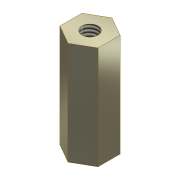
# Autodesk Inventor part: 黄銅スペーサー（六角）_ASB-2613.5E
Saved by Autodesk Inventor 2016 (Build 200138000, 138)
## iProperties
Created: 2016-08-20
Part Number: 黄銅スペーサー（六角）_ASB-2613.5E
Material: 真鍮、ソフト イエロー
Document SubType Name: Modeling
Designer: NN
Mass: 2.07468 g
Surface Area: 3.5973 cm^2
Volume: 0.244944 cm^3
Density: 8.47 g/cm^3
Appearance: ニッケル
Author: NN
Autodesk Inventor part; units mm, degrees
ref_plane "YZ Plane" through (0, 0, 0) normal (1, 0, 0) x (0, 1, 0)
ref_plane "XZ Plane" through (0, 0, 0) normal (0, 1, 0) x (-1, 0, 0)
ref_plane "XY Plane" through (0, 0, 0) normal (0, 0, 1) x (1, 0, 0)
sketch "スケッチ1" plane through (0, 0, 0) normal (0, 0, 1) x (1, 0, 0)
  line L0 (0, 2.8868) -> (2.5, 1.4434)
  line L1 (2.5, 1.4434) -> (2.5, -1.4434)
  line L2 (2.5, -1.4434) -> (0, -2.8868)
  line L3 (0, -2.8868) -> (-2.5, -1.4434)
  line L4 (-2.5, -1.4434) -> (-2.5, 1.4434)
  line L5 (-2.5, 1.4434) -> (0, 2.8868)
  point P0 (0, 0)
  point P1 (0, 0)
  dimension "d0" = 5
  constraints: 12 end point, 1 coincident, 13 other
  measures "d0" distance between parallel lines of L1 L4
extrude "押し出し1" add sketch "スケッチ1" along normal blind 13.5
sketch "スケッチ2" plane through (0, 0, 13.5) normal (0, 0, 1) x (1, 0, 0)
  point P0 (0, 0)
hole "穴1" at (0, 0, 13.5) direction (0, 0, -1) diameter 2.113 depth 7.6 tip angle 118 thread size "M2.6x0.45" class "6H" standard "ISO Metric profile"
sketch "スケッチ3" plane through (0, 0, 0) normal (0, 0, -1) x (-1, 0, 0)
  point P0 (0, 0)
hole "穴2" at (0, 0, 0) direction (0, 0, 1) diameter 2.113 depth 7.6 tip angle 118 thread size "M2.6x0.45" class "6H" standard "ISO Metric profile"
